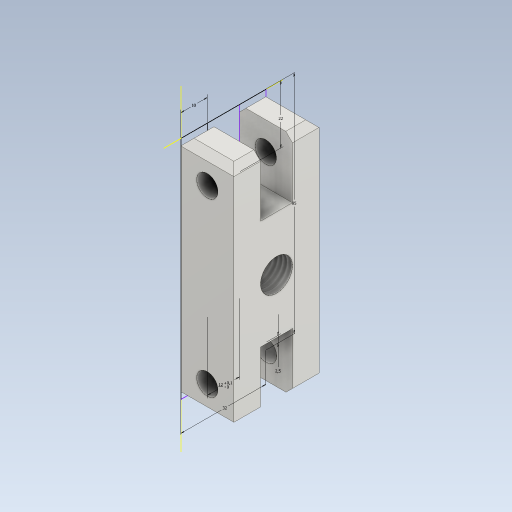
# Autodesk Inventor part: Abzieher_Trägeript
Saved by Autodesk Inventor 2024.3 (Build 283343000, 343)
## iProperties
Created: 2025-08-29
Part Number: Abzieher_Trägeript
Material: 1.0038 S235JR
Document SubType Name: Modeling
Designer: Dickert.Jonas
Density: 7.86 g/cm^3
Appearance: Stahl
Author: Dickert.Jonas
Autodesk Inventor part; units mm, degrees
ref_plane "YZ Plane" through (0, 0, 0) normal (1, 0, 0) x (0, 1, 0)
ref_plane "XZ Plane" through (0, 0, 0) normal (0, 1, 0) x (-1, 0, 0)
ref_plane "XY Plane" through (0, 0, 0) normal (0, 0, 1) x (1, 0, 0)
sketch "Skizze1" plane through (0, 0, 0) normal (1, 0, 0) x (0, 1, 0)
  line L0 (0, -102) -> (0, 17) projected
  line L1 (-6.4, 0) -> (38.4, 0) projected
  line L2 (0, 0) -> (32, 0)
  line L3 (32, 0) -> (32, -85)
  line L4 (32, -85) -> (0, -85)
  line L5 (0, -85) -> (0, 0)
  line L6 (0, 0) -> (10, 0)
  line L7 (10, 0) -> (22, 0)
  line L8 (22, 0) -> (22, -22)
  line L9 (10, -22) -> (10, 0)
  line L10 (10, -85) -> (22.1, -85)
  line L11 (22.1, -85) -> (22.1, -63)
  line L12 (10, -63) -> (10, -85)
  line L13 (22, -22) -> (10, -22)
  line L14 (10, -63) -> (22.1, -63)
  line L15 (32, -2.5) -> (22, -2.5)
  line L16 (10, -2.5) -> (0, -2.5)
  line L17 (32, -85) -> (32, -82.5)
  line L18 (32, -82.5) -> (22.1, -82.5)
  line L19 (10, -82.5) -> (0, -82.5)
  point P0 (16, -42.5)
  dimension "d0" = 32
  dimension "d1" = 85
  dimension "d2" = 10
  dimension "d4" = 22
  dimension "d5" = 12
  dimension "d8" = 2.5
  constraints: 36 end point, 13 point on line, 6 perpendicular, 5 parallel, 4 horizontal
  measures "d0" distance of L4.start L4.end
  measures "d1" distance of L2.end L3.end
  measures "d2" distance of L2.start L6.end
  measures "d4" distance of L7.end L8.end
  measures "d8" distance of L3.end L17.end
extrude "Extrusion2" add sketch "Skizze1" along normal blind 20 contours L0 L19 L12 L4 | L0 L16 L9 L13 L8 L15 L3 L18 L11 L14 L12 L19 | L0 L1 L9 L16 | L11 L18 L3 L4 | L1 L3 L15 L8
chamfer "Fasen5" distance 2.5 angle 45 1 edges at (10, 0, -85) measured on face at (6.6667, 0, -28.3333)
chamfer "Fasen6" distance 2.5 angle 45 1 edges at (10, 32, -85) measured on face at (6.6667, 32, -56.6667)
chamfer "Fasen7" distance 2.5 angle 45 1 edges at (10, 32, 0) measured on face at (13.3333, 32, -55)
chamfer "Fasen8" distance 2.5 angle 45 1 edges at (10, 0, 0) measured on face at (13.3333, 0, -27.5)
hole "Bohrung1" at (0, 16, -42.5) direction (1, 0, 0) diameter 12 end through all
thread "Gewinde1" size "M12x1.75" class "6H" standard "ANSI Metric M Profile" full length
sketch "Skizze2" plane through (0, 32, -82.5) normal (0, 1, 0) x (1, 0, 0)
  line L0 (0, 2.5) -> (0, -19.5) projected
  line L1 (0, 2.5) -> (0, -7.5)
  point P0 (0, -82.5)
  point P1 (10, -7.5)
  point P2 (0, -72.5)
  point P3 (10, -72.047)
  constraints: 2 end point, 1 point on line
hole "Bohrung2" at (10, 32, -75) at (10, 32, -10.453) direction (0, -1, 0) diameter 8 end through all
chamfer "Fasen9" distance 2.5 angle 45 1 edges at (20, 25.75, 0) measured on face at (13.3333, 27, 0)
chamfer "Fasen10" distance 2.5 angle 45 1 edges at (20, 6.25, 0) measured on face at (13.3333, 7.5, 0)
chamfer "Fasen11" distance 2.5 angle 45 1 edges at (20, 25.8, -85) measured on face at (13.3333, 24.5667, -85)
chamfer "Fasen12" distance 2.5 angle 45 1 edges at (20, 6.25, -85) measured on face at (13.3333, 5, -85)
chamfer "Fasen13" distance 2.5 angle 45 1 edges at (0, 25.8, -85) measured on face at (5.8333, 24.5667, -85)
chamfer "Fasen14" distance 2.5 angle 45 1 edges at (0, 6.25, -85) measured on face at (5.8333, 5, -85)
chamfer "Fasen15" distance 2.5 angle 45 1 edges at (0, 25.75, 0) measured on face at (0, 28.6521, -42.2589)
chamfer "Fasen16" distance 2.5 angle 45 1 edges at (0, 6.25, 0) measured on face at (0, 3.3479, -42.7411)
